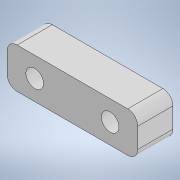
# Autodesk Inventor part: 30_Lasercable_holder_B
Saved by Autodesk Inventor 2022 (Build 260153000, 153)
## iProperties
Created: 2023-01-15
Part Number: 30_Lasercable_holder_B
Material: Generic
Document SubType Name: Modeling
Designer: Max
Density: 1 g/cm^3
Appearance: Default
Author: Max
Autodesk Inventor part; units mm, degrees
ref_plane "YZ Plane" through (0, 0, 0) normal (1, 0, 0) x (0, 1, 0)
ref_plane "XZ Plane" through (0, 0, 0) normal (0, 1, 0) x (-1, 0, 0)
ref_plane "XY Plane" through (0, 0, 0) normal (0, 0, 1) x (1, 0, 0)
sketch "Sketch1" plane through (0, 0, 0) normal (0, 0, 1) x (1, 0, 0)
  line L0 (-13, -4) -> (13, -4)
  line L1 (13, -4) -> (13, 4)
  line L2 (13, 4) -> (-13, 4)
  line L3 (-13, 4) -> (-13, -4)
  line L4 (-13, -4) -> (13, 4) construction
  line L5 (13, -4) -> (-13, 4) construction
  point P0 (0, 0)
  dimension "d0" = 26
  dimension "d1" = 8
  constraints: 12 end point, 2 midpoint, 2 parallel, 1 horizontal, 1 perpendicular
  measures "d0" distance of L2.end L1.end
  measures "d1" distance of L1.end L0.end
extrude "Extrusion1" add sketch "Sketch1" along normal blind 7
sketch "Sketch2" plane through (0, 0, 7) normal (0, 0, 1) x (1, 0, 0)
  line L0 (0, 5.6) -> (0, -5.6) projected
  circle A0 centre (-7.5, 0) radius 1.75
  circle A1 centre (7.5, 0) radius 1.75
  line L1 (-18.2, 0) -> (18.2, 0) projected
  point P0 (0, 0)
  dimension "d4" = 3.5
  dimension "d5" = 15
  constraints: 2 centre point, 1 equal radius, 1 point on line, 1 other
  measures "d4" diameter of A0
  measures "d5" distance of A1.centre A0.centre
extrude "Extrusion2" cut sketch "Sketch2" against normal through all
fillet "Fillet1" radius 2 4 edges at (-13, 4, 3.5) (-13, -4, 3.5) (13, -4, 3.5) (13, 4, 3.5)
body "Solid1"
